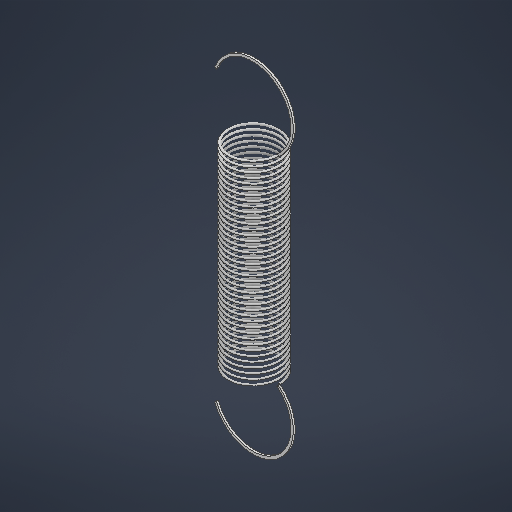
# Autodesk Inventor part: lò xo
Saved by Autodesk Inventor 2027.1 (Build 311270010, 270A)
## iProperties
Created: 2026-08-09
Part Number: lò xo
Material: Generic
Document SubType Name: Sheet Metal
Designer: MSI
Density: 1 g/cm^3
Sheet Metal Rule: Default_mm
Appearance: Default
Author: MSI
Autodesk Inventor part; units mm, degrees
ref_plane "YZ Plane" through (0, 0, 0) normal (1, 0, 0) x (0, 1, 0)
ref_plane "XZ Plane" through (0, 0, 0) normal (0, 1, 0) x (-1, 0, 0)
ref_plane "XY Plane" through (0, 0, 0) normal (0, 0, 1) x (1, 0, 0)
sketch "Sketch1" plane through (0, 0, 0) normal (0, 0, 1) x (1, 0, 0)
  circle A0 centre (2.5, 0) radius 0.1
  line L0 (0, 0) -> (0, 1.121)
  dimension "d0" = 0.2
  dimension "d1" = 2.5
  constraints: 2 end point, 1 centre point, 1 vertical
  measures "d0" diameter of A0
  measures "d1" distance of A0.centre L0.start
coil "Coil1" sketch "Sketch1" operation add axis through (0, 0, 0) along (0, 1, 0) pitch 0.5 turns 40 hand right
sketch "Sketch2" plane through (0, 0, 0) normal (0, 1, 0) x (-1, 0, 0)
  line L0 (-2.6, 0) -> (-2.4, 0) projected
  circle A0 centre (-2.5, 0) radius 0.1
  line L1 (0, 0) -> (-0.8857, 0)
  dimension "d10" = 0.2
  constraints: 2 end point, 1 centre point, 1 horizontal, 1 midpoint
  measures "d10" diameter of A0
sketch "Sketch3" plane through (0, 0, 0) normal (0, 0, 1) x (1, 0, 0)
  circle A0 centre (2.5, 0) radius 0.1 projected
  arc A1 (-3.6215, -4.4696) -> (2.4371, -0.0777) centre (0, -3.0906) ccw
  line L0 (-3.7957, -4.583) -> (-3.6215, -4.4696)
  arc A2 (-3.7957, -4.583) -> (2.5772, 0.0635) centre (0.0316, -3.1386) ccw
  line L1 (0, 10) -> (-6.0861, 10)
  circle A3 centre (2.5, 20) radius 0.1
  arc A4 (2.4371, 20.0777) -> (-3.6215, 24.4696) centre (0, 23.0906) ccw
  line L2 (-3.7957, 24.583) -> (-3.6215, 24.4696)
  arc A5 (2.5772, 19.9365) -> (-3.7957, 24.583) centre (0.0316, 23.1386) ccw
  point P0 (0, 0)
  point P1 (2.6, 0)
  point P2 (0, 20)
  point P3 (2.6, 20)
  constraints: 12 point on circle, 9 symmetric about line, 6 end point, 5 centre point, 1 horizontal, 1 tangent, 3 other
extrude "Extrusion1" add sketch "Sketch3" along normal blind 0.2 contours A0 A2 L0 A1 | A3 A4 L2 A5
equation "\"BendRadius\" = Thickness"
equation "\"BendReliefWidth\" = Thickness"
equation "\"BendReliefDepth\" = 0.5 * Thickness"
equation "\"CornerReliefSize\" = 4 * Thickness"
equation "\"MinimumRemnant\" = 2 * Thickness"
equation "\"TransitionRadius\" = BendRadius"
equation "\"JacobiRadiusSize\" = BendRadius"
equation "\"GapSize\" = Thickness"
equation "\"Thickness\" = 0.5"
body "Solid1"
